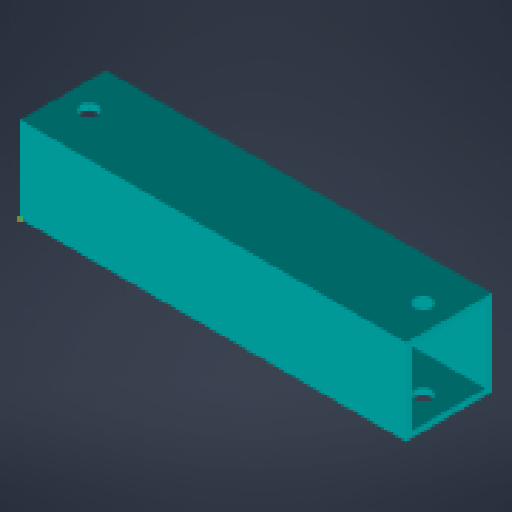
# Autodesk Inventor part: section
Saved by Autodesk Inventor 2024 (Build 280153000, 153)
## iProperties
Created: 2023-04-19
Part Number: section
Material: Типовые
Document SubType Name: Modeling
Designer: user
Density: 1 g/cm^3
Appearance: По умолчанию
Author: user
Autodesk Inventor part; units mm, degrees
ref_plane "YZ Plane" through (0, 0, 0) normal (1, 0, 0) x (0, 1, 0)
ref_plane "XZ Plane" through (0, 0, 0) normal (0, 1, 0) x (-1, 0, 0)
ref_plane "XY Plane" through (0, 0, 0) normal (0, 0, 1) x (1, 0, 0)
sketch "Эскиз2" plane through (0, 0, 0) normal (1, 0, 0) x (0, 1, 0)
  line L0 (0, 0) -> (20, 0)
  line L1 (20, 0) -> (20, 20)
  line L2 (20, 20) -> (0, 20)
  line L3 (0, 20) -> (0, 0)
  line L4 (18.5, 18.5) -> (1.5, 18.5)
  line L5 (1.5, 18.5) -> (1.5, 1.5)
  line L6 (1.5, 1.5) -> (18.5, 1.5)
  line L7 (18.5, 1.5) -> (18.5, 18.5)
  point P0 (10, 18.5)
  point P1 (10, 20)
  point P2 (18.5, 10)
  point P3 (20, 10)
  dimension "d0" = 20
  dimension "d1" = 1.5
  constraints: 16 end point, 4 midpoint, 4 parallel, 4 perpendicular, 2 horizontal, 1 horizontal alignment, 1 vertical alignment
  measures "d0" distance of L0.end L1.end
  measures "d1" horizontal distance of L1.end L4.start
extrude "Выдавливание1" add sketch "Эскиз2" along normal blind 90
sketch "Эскиз3" plane through (0, 0, 20) normal (0, 0, 1) x (1, 0, 0)
  circle A0 centre (6, 10) radius 2
  circle A1 centre (84, 10) radius 2
  line L0 (90, 20) -> (90, 0) projected
  line L1 (0, 20) -> (0, 0) projected
  point P0 (90, 10)
  point P1 (0, 10)
  point P2 (90, 10)
  point P3 (0, 10)
  dimension "d6" = 6
  dimension "d7" = 6
  dimension "d10" = 4
  constraints: 4 midpoint, 2 centre point, 2 horizontal alignment, 1 equal radius
  measures "d6" distance of point (90, 10) A1.centre
  measures "d7" distance of point (0, 10) A0.centre
  measures "d10" diameter of A1
extrude "Выдавливание2" cut sketch "Эскиз3" against normal through all
equation "\"d7\" = d6"
